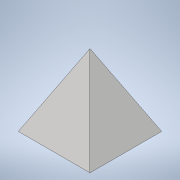
# Autodesk Inventor part: PyramidPiece-ver1-1111-2021
Saved by Autodesk Inventor 2021 (Build 250183000, 183)
## iProperties
Created: 2016-01-22
Part Number: PyramidPiece-ver1-1111-2021
Material: Generic
Document SubType Name: Modeling
Designer: anishfl
Density: 1 g/cm^3
Appearance: Default
Author: anishfl
Autodesk Inventor part; units mm, degrees
sketch "Sketch1" plane through (0, 0, 0) normal (0, 1, 0) x (-1, 0, 0)
  line L0 (11.0913, -5.6727) -> (4.7413, -5.6727)
  line L1 (4.7413, -5.6727) -> (4.7413, -12.0227)
  line L2 (4.7413, -12.0227) -> (11.0913, -12.0227)
  line L3 (11.0913, -12.0227) -> (11.0913, -5.6727)
  point P0 (0, 0)
  dimension "d0" = 6.35
  dimension "d1" = 6.35
  constraints: 8 end point, 2 parallel, 1 horizontal, 1 perpendicular
  measures "d0" distance of L2.end L0.start
  measures "d1" distance of L1.end L2.end
extrude "Extrusion1" add sketch "Sketch1" along normal blind 6.35
sketch "Sketch2" plane through (0, 6.35, 0) normal (0, 1, 0) x (1, 0, 0)
  line L0 (-11.0913, 5.6727) -> (-4.7413, 5.6727) projected
  line L1 (-7.9163, 5.6727) -> (-7.9163, 31.288)
  line L2 (-11.0913, 12.0227) -> (-11.0913, 5.6727) projected
  line L3 (-11.0913, 8.8477) -> (-4.7413, 8.8477)
  line L4 (-4.7413, 5.6727) -> (-4.7413, 12.0227) projected
  point P0 (0, 0)
  constraints: 4 end point, 3 midpoint, 1 vertical
ref_plane "Work Plane1" through (-11.0913, 6.35, -8.8477) normal (0, -0.4472, -0.8944) x (1, 0, 0)
ref_plane "Work Plane2" through (-7.9163, 6.35, -5.6727) normal (-0.8944, -0.4472, 0) x (0, 0, -1)
sketch "Sketch3" plane through (-7.9163, 6.35, -5.6727) normal (-0.8944, -0.4472, 0) x (0, 0, -1)
  circle A0 centre (4.2078, 1.1693) radius 62.6047
  point P0 (-5.6727, 9.2199)
  constraints: 1 centre point
extrude "Extrusion2" cut sketch "Sketch3" against normal blind 6.35
sketch "Sketch4" plane through (-11.0913, 6.35, -8.8477) normal (0, -0.4472, -0.8944) x (1, 0, 0)
  circle A0 centre (3.6539, 12.2089) radius 78.9893
  point P0 (11.0913, 9.6364)
  constraints: 1 centre point
extrude "Extrusion3" cut sketch "Sketch4" against normal blind 6.35
ref_plane "Work Plane3" through (-7.9163, 6.35, -5.6727) normal (-0.8944, 0.4472, 0) x (0, 0, -1)
sketch "Sketch5" plane through (-7.9163, 6.35, -5.6727) normal (-0.8944, 0.4472, 0) x (0, 0, -1)
  circle A0 centre (14.7734, 12.1787) radius 25.4
  point P0 (-5.6727, 2.1393)
  dimension "d14" = 50.8
  constraints: 1 centre point
  measures "d14" diameter of A0
extrude "Extrusion4" cut sketch "Sketch5" along normal blind 6.35
ref_plane "Work Plane4" through (-11.0913, 6.35, -8.8477) normal (0, 0.4472, -0.8944) x (1, 0, 0)
sketch "Sketch6" plane through (-11.0913, 6.35, -8.8477) normal (0, 0.4472, -0.8944) x (1, 0, 0)
  circle A0 centre (11.0913, 15.7599) radius 33.5156
  point P0 (11.0913, 1.7228)
  constraints: 1 centre point
extrude "Extrusion5" cut sketch "Sketch6" along normal blind 6.35
body "Solid1"
